Autodesk Inventor part; units mm, degrees
(part 2 of 2)
  line L172 (15.8451, 2.3922) -> (13.6033, 2.3922)
  line L173 (13.6033, 2.3922) -> (13.6033, 2.889)
  spline S178 degree 2 poles (13.6033, 2.889) (13.8875, 3.1164) (14.3423, 3.5168) (14.5129, 3.6973) knots 0 0 0 1 2 2 2
  spline S179 degree 2 poles (14.5129, 3.6973) (14.7378, 3.9321) (14.938, 4.2905) (14.938, 4.4783) knots 0 0 0 1 2 2 2
  spline S180 degree 2 poles (14.938, 4.4783) (14.938, 4.6909) (14.6834, 4.9183) (14.456, 4.9183) knots 0 0 0 1 2 2 2
  spline S181 degree 2 poles (14.456, 4.9183) (14.3398, 4.9183) (14.1322, 4.8614) (14.0259, 4.8169) knots 0 0 0 1 2 2 2
  spline S182 degree 2 poles (14.0259, 4.8169) (13.9221, 4.77) (13.7738, 4.6711) (13.7368, 4.6464) knots 0 0 0 1 2 2 2
  line L174 (13.7368, 4.6464) -> (13.6774, 4.6464)
  line L175 (13.6774, 4.6464) -> (13.6774, 5.3113)
  spline S183 degree 2 poles (13.6774, 5.3113) (13.806, 5.373) (14.3547, 5.5016) (14.6092, 5.5016) knots 0 0 0 1 2 2 2
  spline S184 degree 2 poles (14.6092, 5.5016) (15.153, 5.5016) (15.7116, 5.0171) (15.7116, 4.5796) knots 0 0 0 1 2 2 2
  spline S185 degree 2 poles (15.7116, 4.5796) (15.7116, 4.3102) (15.457, 3.7912) (15.1629, 3.4946) knots 0 0 0 1 2 2 2
  spline S186 degree 2 poles (15.1629, 3.4946) (14.9775, 3.3117) (14.629, 3.0275) (14.5524, 2.9681) knots 0 0 0 1 2 2 2
  line L176 (14.5524, 2.9681) -> (15.8451, 2.9681)
  line L177 (15.8451, 2.9681) -> (15.8451, 2.3922)
  line L178 (18.554, 3.1041) -> (18.1412, 3.1041)
  line L179 (18.1412, 3.1041) -> (18.1412, 2.3848)
  line L180 (18.1412, 2.3848) -> (17.4022, 2.3848)
  line L181 (17.4022, 2.3848) -> (17.4022, 3.1041)
  line L182 (17.4022, 3.1041) -> (16.0576, 3.1041)
  line L183 (16.0576, 3.1041) -> (16.0576, 3.6726)
  line L184 (16.0576, 3.6726) -> (17.3775, 5.4422)
  line L185 (17.3775, 5.4422) -> (18.1412, 5.4422)
  line L186 (18.1412, 5.4422) -> (18.1412, 3.6528)
  line L187 (18.1412, 3.6528) -> (18.554, 3.6528)
  line L188 (18.554, 3.6528) -> (18.554, 3.1041)
  line L189 (17.4022, 3.6528) -> (17.4022, 4.6909)
  line L190 (17.4022, 4.6909) -> (16.6286, 3.6528)
  line L191 (16.6286, 3.6528) -> (17.4022, 3.6528)
  line L192 (21.0652, 4.6933) -> (20.2396, 2.3922)
  line L193 (20.2396, 2.3922) -> (19.4561, 2.3922)
  line L194 (19.4561, 2.3922) -> (18.638, 4.6933)
  line L195 (18.638, 4.6933) -> (19.3919, 4.6933)
  line L196 (19.3919, 4.6933) -> (19.8615, 3.1733)
  line L197 (19.8615, 3.1733) -> (20.3261, 4.6933)
  line L198 (20.3261, 4.6933) -> (21.0652, 4.6933)
  line L199 (22.647, 3.4551) -> (21.2901, 3.4551)
  line L200 (21.2901, 3.4551) -> (21.2901, 4.0235)
  line L201 (21.2901, 4.0235) -> (22.647, 4.0235)
  line L202 (22.647, 4.0235) -> (22.647, 3.4551)
  spline S187 degree 2 poles (25.3559, 3.4254) (25.3559, 3.1856) (25.1928, 2.7803) (25.0321, 2.6345) knots 0 0 0 1 2 2 2
  spline S188 degree 2 poles (25.0321, 2.6345) (24.8715, 2.4886) (24.4315, 2.328) (24.1102, 2.328) knots 0 0 0 1 2 2 2
  spline S189 degree 2 poles (24.1102, 2.328) (23.7691, 2.3305) (23.2798, 2.4417) (23.1191, 2.5134) knots 0 0 0 1 2 2 2
  line L203 (23.1191, 2.5134) -> (23.1191, 3.1782)
  line L204 (23.1191, 3.1782) -> (23.1883, 3.1782)
  spline S190 degree 2 poles (23.1883, 3.1782) (23.2476, 3.1461) (23.391, 3.0621) (23.5071, 3.0176) knots 0 0 0 1 2 2 2
  spline S191 degree 2 poles (23.5071, 3.0176) (23.6159, 2.9756) (23.8408, 2.9187) (23.9768, 2.9187) knots 0 0 0 1 2 2 2
  spline S192 degree 2 poles (23.9768, 2.9187) (24.0954, 2.9187) (24.3722, 2.978) (24.4563, 3.0571) knots 0 0 0 1 2 2 2
  spline S193 degree 2 poles (24.4563, 3.0571) (24.518, 3.1189) (24.5872, 3.2697) (24.5872, 3.3957) knots 0 0 0 1 2 2 2
  spline S194 degree 2 poles (24.5872, 3.3957) (24.5872, 3.5045) (24.4983, 3.6577) (24.4266, 3.7047) knots 0 0 0 1 2 2 2
  spline S195 degree 2 poles (24.4266, 3.7047) (24.3228, 3.7739) (24.0262, 3.8134) (23.9199, 3.8134) knots 0 0 0 1 2 2 2
  spline S196 degree 2 poles (23.9199, 3.8134) (23.7518, 3.8134) (23.433, 3.7591) (23.3168, 3.7294) knots 0 0 0 1 2 2 2
  line L205 (23.3168, 3.7294) -> (23.2501, 3.7294)
  line L206 (23.2501, 3.7294) -> (23.2501, 5.4422)
  line L207 (23.2501, 5.4422) -> (25.2719, 5.4422)
  line L208 (25.2719, 5.4422) -> (25.2719, 4.8664)
  line L209 (25.2719, 4.8664) -> (23.9743, 4.8664)
  line L210 (23.9743, 4.8664) -> (23.9743, 4.3597)
  spline S197 degree 2 poles (23.9743, 4.3597) (24.0361, 4.3646) (24.2066, 4.3696) (24.2536, 4.3696) knots 0 0 0 1 2 2 2
  spline S198 degree 2 poles (24.2536, 4.3696) (24.4736, 4.3696) (24.8443, 4.2806) (24.9901, 4.1891) knots 0 0 0 1 2 2 2
  spline S199 degree 2 poles (24.9901, 4.1891) (25.1631, 4.0754) (25.3559, 3.6973) (25.3559, 3.4254) knots 0 0 0 1 2 2 2
  line L211 (27.9734, 4.6933) -> (27.1479, 2.3922)
  line L212 (27.1479, 2.3922) -> (26.3644, 2.3922)
  line L213 (26.3644, 2.3922) -> (25.5462, 4.6933)
  line L214 (25.5462, 4.6933) -> (26.3001, 4.6933)
  line L215 (26.3001, 4.6933) -> (26.7697, 3.1733)
  line L216 (26.7697, 3.1733) -> (27.2344, 4.6933)
  line L217 (27.2344, 4.6933) -> (27.9734, 4.6933)
  spline S200 degree 2 poles (31.6759, 3.3166) (31.6759, 3.0917) (31.5103, 2.7234) (31.3496, 2.5949) knots 0 0 0 1 2 2 2
  spline S201 degree 2 poles (31.3496, 2.5949) (31.189, 2.4664) (30.7515, 2.328) (30.4376, 2.328) knots 0 0 0 1 2 2 2
  spline S202 degree 2 poles (30.4376, 2.328) (30.0817, 2.328) (29.5725, 2.4466) (29.4119, 2.5208) knots 0 0 0 1 2 2 2
  line L218 (29.4119, 2.5208) -> (29.4119, 3.1832)
  line L219 (29.4119, 3.1832) -> (29.486, 3.1832)
  spline S203 degree 2 poles (29.486, 3.1832) (29.6541, 3.0769) (30.1064, 2.9187) (30.2943, 2.9187) knots 0 0 0 1 2 2 2
  spline S204 degree 2 poles (30.2943, 2.9187) (30.4055, 2.9187) (30.665, 2.9583) (30.754, 3.0225) knots 0 0 0 1 2 2 2
  spline S205 degree 2 poles (30.754, 3.0225) (30.8232, 3.0744) (30.9072, 3.2252) (30.9072, 3.3611) knots 0 0 0 1 2 2 2
  spline S206 degree 2 poles (30.9072, 3.3611) (30.9072, 3.4971) (30.7886, 3.6429) (30.6897, 3.6775) knots 0 0 0 1 2 2 2
  spline S207 degree 2 poles (30.6897, 3.6775) (30.5909, 3.7121) (30.3165, 3.7195) (30.2102, 3.7195) knots 0 0 0 1 2 2 2
  line L220 (30.2102, 3.7195) -> (30.0792, 3.7195)
  line L221 (30.0792, 3.7195) -> (30.0792, 4.2559)
  line L222 (30.0792, 4.2559) -> (30.2003, 4.2559)
  spline S208 degree 2 poles (30.2003, 4.2559) (30.3387, 4.2559) (30.5736, 4.2806) (30.6551, 4.3177) knots 0 0 0 1 2 2 2
  spline S209 degree 2 poles (30.6551, 4.3177) (30.7367, 4.3572) (30.8281, 4.4956) (30.8281, 4.6143) knots 0 0 0 1 2 2 2
  spline S210 degree 2 poles (30.8281, 4.6143) (30.8281, 4.7082) (30.7416, 4.8243) (30.6798, 4.8565) knots 0 0 0 1 2 2 2
  spline S211 degree 2 poles (30.6798, 4.8565) (30.6057, 4.8935) (30.408, 4.9183) (30.3387, 4.9183) knots 0 0 0 1 2 2 2
  spline S212 degree 2 poles (30.3387, 4.9183) (30.2275, 4.9183) (29.9927, 4.8664) (29.884, 4.8243) knots 0 0 0 1 2 2 2
  spline S213 degree 2 poles (29.884, 4.8243) (29.7975, 4.7922) (29.6096, 4.6884) (29.5651, 4.6612) knots 0 0 0 1 2 2 2
  line L223 (29.5651, 4.6612) -> (29.5009, 4.6612)
  line L224 (29.5009, 4.6612) -> (29.5009, 5.3137)
  spline S214 degree 2 poles (29.5009, 5.3137) (29.659, 5.3805) (30.1929, 5.5065) (30.4722, 5.5065) knots 0 0 0 1 2 2 2
  spline S215 degree 2 poles (30.4722, 5.5065) (30.7441, 5.5065) (31.1445, 5.4126) (31.2854, 5.3211) knots 0 0 0 1 2 2 2
  spline S216 degree 2 poles (31.2854, 5.3211) (31.4411, 5.2247) (31.5968, 4.9281) (31.5968, 4.7428) knots 0 0 0 1 2 2 2
  spline S217 degree 2 poles (31.5968, 4.7428) (31.5968, 4.4808) (31.2953, 4.0903) (31.0481, 4.0334) knots 0 0 0 1 2 2 2
  line L225 (31.0481, 4.0334) -> (31.0481, 4.0038)
  spline S218 degree 2 poles (31.0481, 4.0038) (31.1569, 3.9889) (31.3645, 3.9098) (31.4633, 3.8209) knots 0 0 0 1 2 2 2
  spline S219 degree 2 poles (31.4633, 3.8209) (31.5548, 3.7418) (31.6759, 3.4897) (31.6759, 3.3166) knots 0 0 0 1 2 2 2
  line L226 (31.8613, 2.3922) -> (32.8919, 5.4422)
  line L227 (32.8919, 5.4422) -> (33.7274, 5.4422)
  line L228 (33.7274, 5.4422) -> (34.758, 2.3922)
  line L229 (34.758, 2.3922) -> (33.9696, 2.3922)
  line L230 (33.9696, 2.3922) -> (33.7793, 3.0151)
  line L231 (33.7793, 3.0151) -> (32.8203, 3.0151)
  line L232 (32.8203, 3.0151) -> (32.6275, 2.3922)
  line L233 (32.6275, 2.3922) -> (31.8613, 2.3922)
  line L234 (33.6112, 3.5687) -> (33.2998, 4.5772)
  line L235 (33.2998, 4.5772) -> (32.9859, 3.5687)
  line L236 (32.9859, 3.5687) -> (33.6112, 3.5687)
  point P0 (24.6, -0.25)
  constraints: 2 other
extrude "Extrusion14" cut sketch "Sketch17" against normal blind 0.6
body "Solid1"
